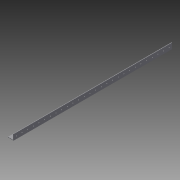
# Autodesk Inventor part: bumper_angle
Saved by Autodesk Inventor 2015 SP1 (Build 190203100, 203)
## iProperties
Created: 2014-12-23
Part Number: bumper_angle
Material: Generic
Document SubType Name: Modeling
Designer: Jarod
Density: 1 g/cm^3
Appearance: Default
Author: Jarod
Autodesk Inventor part; units mm, degrees
ref_plane "YZ Plane" through (0, 0, 0) normal (1, 0, 0) x (0, 1, 0)
ref_plane "XZ Plane" through (0, 0, 0) normal (0, 1, 0) x (-1, 0, 0)
ref_plane "XY Plane" through (0, 0, 0) normal (0, 0, 1) x (1, 0, 0)
sketch "Sketch1" plane through (0, 0, 0) normal (0, 0, 1) x (1, 0, 0)
  line L0 (0, 0) -> (-25.4, 0)
  line L1 (-25.4, 0) -> (-25.4, 2.286)
  line L2 (-25.4, 2.286) -> (0, 2.286)
  line L3 (0, 2.286) -> (0, 0)
  line L4 (0, 0) -> (-2.286, 0)
  line L5 (-2.286, 0) -> (-2.286, 25.4)
  line L6 (-2.286, 25.4) -> (0, 25.4)
  line L7 (0, 25.4) -> (0, 0)
  dimension "d0" = 25.4
  dimension "d1" = 2.286
  dimension "d2" = 2.286
  dimension "d3" = 25.4
  constraints: 16 end point, 4 parallel, 2 horizontal, 2 perpendicular
  measures "d0" distance of L1.end L2.end
  measures "d1" distance of L0.end L1.end
  measures "d2" distance of L5.end L6.end
  measures "d3" distance of L4.end L5.end
extrude "Extrusion1" add sketch "Sketch1" along normal blind 711.2
sketch "Sketch2" plane through (-25.4, 0, 0) normal (0, -1, 0) x (1, 0, 0)
  line L0 (0, 0) -> (25.4, 0) projected
  line L1 (25.4, 0) -> (25.4, 711.2) projected
  line L2 (0, 711.2) -> (25.4, 711.2) projected
  line L3 (0, 0) -> (0, 711.2) projected
  point P0 (12.7, 12.7)
  dimension "d6" = 12.7
  dimension "d7" = 12.7
  measures "d6" distance from line of L1 point (12.7, 12.7)
  measures "d7" distance from line of L0 point (12.7, 12.7)
hole "Hole1" at (-12.7, 0, 12.7) direction (0, 1, 0) diameter 3.9688 end through all
pattern_linear "Rectangular Pattern1" count 28 spacing 25.4 along (0, 0, 1) of "Hole1"
sketch "Sketch3" plane through (0, 0, 0) normal (1, 0, 0) x (0, 0, -1)
  line L0 (-711.2, 0) -> (-711.2, 25.4) projected
  line L1 (0, 0) -> (-711.2, 0) projected
  line L2 (0, 0) -> (0, 25.4) projected
  line L3 (0, 25.4) -> (-711.2, 25.4) projected
  point P0 (-12.7, 12.7)
  dimension "d18" = 12.7
  dimension "d19" = 12.7
  measures "d18" distance from line of L1 point (-12.7, 12.7)
  measures "d19" distance from line of L2 point (-12.7, 12.7)
hole "Hole2" at (0, 12.7, 12.7) direction (-1, 0, 0) diameter 3.9688 end through all
pattern_linear "Rectangular Pattern2" count 28 spacing 25.4 along (0, 0, 1) of "Hole2"
body "Solid1"
